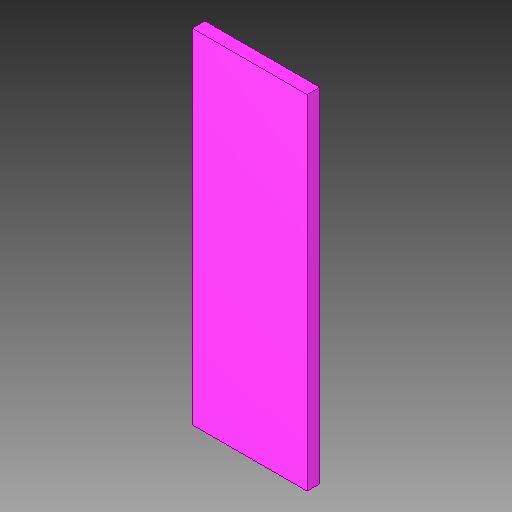
# Autodesk Inventor part: SICHERUNG
Saved by Autodesk Inventor 2017 (Build 210142000, 142)
## iProperties
Created: 2019-06-13
Part Number: SICHERUNG
Material: Generic
Document SubType Name: Modeling
Designer: Marc
Density: 1 g/cm^3
Appearance: SICHERUNG, SICHERUNG
Author: Marc
Autodesk Inventor part; units mm, degrees
ref_plane "YZ Plane" through (0, 0, 0) normal (1, 0, 0) x (0, 1, 0)
ref_plane "XZ Plane" through (0, 0, 0) normal (0, 1, 0) x (-1, 0, 0)
ref_plane "XY Plane" through (0, 0, 0) normal (0, 0, 1) x (1, 0, 0)
sketch "SICHERUNG, SICHERUNG_59" plane through (0, 0, 0) normal (0, 0, 1) x (1, 0, 0)
  line L0 (-4.5, 13.55) -> (4.5635, 13.55)
  line L1 (4.5635, 13.55) -> (4.5635, -13.55)
  line L2 (4.5635, -13.55) -> (-4.5, -13.55)
  line L3 (-4.5, -13.55) -> (-4.5, 13.55)
  constraints: 8 end point
extrude "Extrusion1" add sketch "SICHERUNG, SICHERUNG_59" along normal blind 1
body "Solid1"
